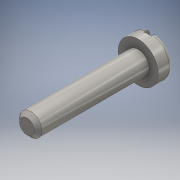
# Autodesk Inventor part: machineScrew3x10
Saved by Autodesk Inventor 2016 (Build 200138000, 138)
## iProperties
Created: 2016-06-30
Part Number: machineScrew3x10
Material: Stainless Steel
Document SubType Name: Modeling
Designer: hesaon
Density: 8 g/cm^3
Appearance: Semi-Polished
Author: hesaon
Autodesk Inventor part; units mm, degrees
ref_plane "YZ Plane" through (0, 0, 0) normal (1, 0, 0) x (0, 1, 0)
ref_plane "XZ Plane" through (0, 0, 0) normal (0, 1, 0) x (-1, 0, 0)
ref_plane "XY Plane" through (0, 0, 0) normal (0, 0, 1) x (1, 0, 0)
sketch "Sketch1" plane through (0, 0, 0) normal (0, 1, 0) x (-1, 0, 0)
  circle A0 centre (0, 0) radius 2.7
  dimension "headDiameter" = 5.4
  constraints: 1 centre point, 1 coincident
  measures "headDiameter" diameter of A0
extrude "Extrusion1" add sketch "Sketch1" along normal blind 2
sketch "Sketch2" plane through (0, 2, 0) normal (0, 1, 0) x (1, 0, 0)
  line L0 (0.5, -2.7) -> (-0.5, -2.7)
  line L1 (-0.5, -2.7) -> (-0.5, 2.7)
  line L2 (-0.5, 2.7) -> (0.5, 2.7)
  line L3 (0.5, 2.7) -> (0.5, -2.7)
  line L4 (0.5, -2.7) -> (-0.5, 2.7) construction
  line L5 (-0.5, -2.7) -> (0.5, 2.7) construction
  point P0 (0, 0)
  dimension "d3" = 1
  dimension "d4" = 5.4
  constraints: 12 end point, 2 midpoint, 2 parallel, 1 horizontal, 1 perpendicular
  measures "d3" distance of L1.end L2.end
  measures "d4" distance of L0.end L1.end
extrude "Extrusion2" cut sketch "Sketch2" against normal blind 0.75
sketch "Sketch3" plane through (0, 0, 0) normal (0, -1, 0) x (1, 0, 0)
  circle A0 centre (0, 0) radius 1.5
  dimension "d7" = 3
  constraints: 1 centre point, 1 coincident
  measures "d7" diameter of A0
extrude "Extrusion3" add sketch "Sketch3" along normal blind 15
chamfer "Chamfer1" distance 0.5 angle 45 1 edges at (-1.5, -15, 0)
fillet "Fillet1" radius 0.5 3 edges at (-2.0785, 2, 1.7234) (-2.0785, 2, -1.7234) (2.7, 2, 0)
equation "\"d4\" = headDiameter"
body "Solid1"
